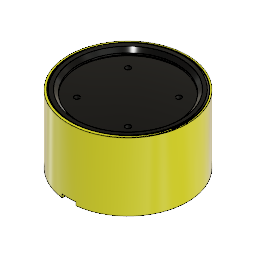
Rotating ROV thruster base v10 (Autodesk Fusion 360 archive; units mm, degrees)
design "Rotating ROV thruster base" references "Servo sg90"
Autodesk Fusion 360 part; units mm, degrees
note: some values were not read from the file. Set by a fixed rule: which face or edge a step refers to.
sketch "Sketch1" plane through (0, 0, 0) normal (0, 0, 1) x (1, 0, 0)
  line L0 (-15, 15) -> (15, 15) construction
  line L1 (15, 15) -> (15, -15) construction
  line L2 (15, -15) -> (-15, -15) construction
  line L3 (-15, -15) -> (-15, 15) construction
  line L4 (-15, 15) -> (15, -15) construction
  line L5 (15, 15) -> (-15, -15) construction
  circle A0 centre (15, 15) radius 1.5
  circle A1 centre (-15, 15) radius 1.5
  circle A2 centre (-15, -15) radius 1.5
  circle A3 centre (15, -15) radius 1.5
  line L6 (-20, 20) -> (20, 20)
  line L7 (20, 20) -> (20, -20)
  line L8 (20, -20) -> (-20, -20)
  line L9 (-20, -20) -> (-20, 20)
  line L10 (-20, 20) -> (20, -20) construction
  line L11 (20, 20) -> (-20, -20) construction
  circle A4 centre (-15, 15) radius 3
  circle A5 centre (15, 15) radius 3
  circle A6 centre (-15, -15) radius 3
  circle A7 centre (15, -15) radius 3
  circle A8 centre (0, 0) radius 35
  dimension "d1" = 30
  dimension "d2" = 30
  dimension "d3" = 3
  dimension "d4" = 3
  dimension "d5" = 3
  dimension "d6" = 3
  dimension "d7" = 40
  dimension "d8" = 40
  dimension "d11" = 6
  dimension "d12" = 6
  dimension "d13" = 6
  dimension "d14" = 6
  constraint perpendicular L0 L1
  constraint parallel L0 L2
  constraint parallel L1 L3
  constraint horizontal L0
  constraint coincident L4 A8.centre
  constraint coincident L5 A8.centre
  constraint coincident A8.centre origin
  constraint coincident L0.end L1.start
  constraint coincident L0.start L3.end
  constraint coincident L2.end L3.start
  constraint coincident L1.end L2.start
  constraint perpendicular L6 L7
  constraint parallel L6 L8
  constraint parallel L7 L9
  constraint horizontal L6
  constraint coincident L10 A8.centre
  constraint coincident L11 A8.centre
  constraint concentric A1 A4
  constraint concentric A0 A5
  constraint concentric A2 A6
  constraint concentric A3 A7
  measures "d1" distance of L0.end L1.end
  measures "d2" distance of L1.end L2.end
  measures "d3" diameter of A0
  measures "d4" diameter of A1
  measures "d5" diameter of A2
  measures "d6" diameter of A3
  measures "d7" distance of L7.end L8.end
  measures "d8" distance of L6.end L7.end
  measures "d11" diameter of A4
  measures "d12" diameter of A5
  measures "d13" diameter of A6
  measures "d14" diameter of A7
extrude "Extrude3" add sketch "Sketch1" along normal blind 16 contours L6 L7 L8 L9 makes body 1
extrude "Extrude4" add sketch "Sketch1" along normal blind 2 contours A4 | A5 | A6 | A7 bodies 1
sketch "Sketch2" plane through (0, 0, 16) normal (0, 0, 1) x (-1, 0, 0)
  circle A0 centre (15, 15) radius 3
  circle A1 centre (-15, -15) radius 3
  circle A2 centre (-15, 15) radius 3
  circle A3 centre (15, -15) radius 3
  line L0 (20, 20) -> (-20, 20)
  line L1 (-20, 20) -> (-20, -20)
  line L2 (-20, -20) -> (20, -20)
  line L3 (20, -20) -> (20, 20)
  line L4 (6.225, 16.425) -> (-6.225, 16.425)
  line L5 (-6.225, 16.425) -> (-6.225, -6.425)
  line L6 (-6.225, -6.425) -> (6.225, -6.425)
  line L7 (6.225, -6.425) -> (6.225, 16.425)
  circle A4 centre (0, -8.925) radius 1.5
  line L8 (-20, 0) -> (-2.5, 0)
  line L9 (-6.225, 5) -> (6.225, 5) construction
  circle A5 centre (0, 18.925) radius 1.5
  dimension "d21" = 12.45
  dimension "d22" = 22.85
  dimension "d25" = 3
  constraint perpendicular L4 L5
  constraint parallel L4 L6
  constraint parallel L5 L7
  constraint horizontal L4
  constraint midpoint L5 L9.start
  constraint midpoint L7 L9.end
  constraint symmetric A4 L9 A5
  measures "d21" distance of L5.end L6.end
  measures "d22" distance of L4.end L5.end
  measures "d25" diameter of A4
extrude "Extrude5" cut sketch "Sketch2" against normal up to surface (16 mm away) contours L4 L5 L6 L7 bodies 1
sketch "Sketch3" plane through (0, 20, 0) normal (0, 1, 0) x (-1, 0, 0)
  line L0 (-20, 0) -> (20, 0)
  line L1 (20, 0) -> (20, 16)
  line L2 (20, 16) -> (-20, 16)
  line L3 (-20, 16) -> (-20, 0)
  line L4 (-4, 2) -> (4, 2)
  line L5 (4, 2) -> (4, -2)
  line L6 (4, -2) -> (-4, -2)
  line L7 (-4, -2) -> (-4, 2)
  line L8 (-4, 2) -> (4, -2) construction
  line L9 (4, 2) -> (-4, -2) construction
  constraint perpendicular L4 L5
  constraint parallel L4 L6
  constraint parallel L5 L7
  constraint horizontal L4
  constraint coincident L8 origin
  constraint coincident L9 origin
extrude "Extrude7" cut sketch "Sketch2" against normal blind 10 contours L0 A5 | L0 A5 | A4 bodies 1
extrude "Extrude8" add sketch "Sketch1" along normal blind 16 contours A8 bodies 1
extrude "Extrude6" cut sketch "Sketch3" along normal blind 30 and the other way blind 65 contours L0 L4 L5 L7 bodies 1
sketch "Sketch4" plane through (0, 0, 16) normal (0, 0, 1) x (-1, 0, 0)
  circle A0 centre (0, 0) radius 35
  circle A1 centre (0, -8.925) radius 1.5
  line L0 (6.225, -6.425) -> (-6.225, -6.425)
  line L1 (-6.225, -6.425) -> (-6.225, 16.425)
  line L2 (-6.225, 16.425) -> (6.225, 16.425)
  line L3 (6.225, 16.425) -> (6.225, -6.425)
  circle A2 centre (15, 15) radius 3
  circle A3 centre (-15, 15) radius 3
  circle A4 centre (-15, -15) radius 3
  circle A5 centre (15, -15) radius 3
  circle A6 centre (0, 0) radius 33
  arc A7 (-1.0461, 20) -> (1.0461, 20) centre (0, 18.925) ccw
  line L4 (-1.0461, 20) -> (1.0461, 20)
  dimension "d34" = -2
extrude "Extrude9" add sketch "Sketch4" along normal blind 20 contours A0 bodies 1
sketch "Sketch6" plane through (0, 0, 16) normal (0, 0, 1) x (-1, 0, 0)
  circle A0 centre (0, 0) radius 33
  circle A1 centre (0, -8.925) radius 1.5
  line L0 (6.225, -6.425) -> (-6.225, -6.425)
  line L1 (-6.225, -6.425) -> (-6.225, 16.425)
  line L2 (-6.225, 16.425) -> (6.225, 16.425)
  line L3 (6.225, 16.425) -> (6.225, -6.425)
  circle A2 centre (15, 15) radius 3
  circle A3 centre (-15, 15) radius 3
  circle A4 centre (-15, -15) radius 3
  circle A5 centre (15, -15) radius 3
  line L4 (6.225, -11.775) -> (-6.225, -11.775)
  line L5 (-6.225, -11.775) -> (-6.225, 20.475)
  line L6 (-6.225, 20.475) -> (6.225, 20.475)
  line L7 (6.225, 20.475) -> (6.225, -11.775)
  arc A6 (-1.0461, 20) -> (1.0461, 20) centre (0, 18.925) ccw
  line L8 (-1.0461, 20) -> (1.0461, 20)
  point P0 (6.225, -11.775)
  point P1 (-6.225, 20.475)
  constraint horizontal L4
  constraint vertical L5
  constraint horizontal L6
  constraint vertical L7
  constraint coincident P1 L5.end
  constraint coincident P0 L4.start
extrude "Extrude11" add sketch "Sketch6" along normal blind 11 contours A0 bodies 1
sketch "Sketch8" plane through (0, 0, 27) normal (0, 0, 1) x (-1, 0, 0)
  circle A0 centre (15, -15) radius 3
  circle A1 centre (-15, 15) radius 3
  circle A2 centre (-15, -15) radius 3
  line L0 (-6.225, 20.475) -> (6.225, 20.475)
  line L1 (6.225, 20.475) -> (6.225, -11.775)
  line L2 (6.225, -11.775) -> (-6.225, -11.775)
  line L3 (-6.225, -11.775) -> (-6.225, 20.475)
  circle A3 centre (15, 15) radius 3
  circle A4 centre (0, 0) radius 33
  circle A5 centre (0, 0) radius 30
  line L4 (13.2679, -12) -> (11.5359, -15)
  line L5 (11.5359, -15) -> (13.2679, -18)
  line L6 (13.2679, -18) -> (16.7321, -18)
  line L7 (16.7321, -18) -> (18.4641, -15)
  line L8 (18.4641, -15) -> (16.7321, -12)
  line L9 (16.7321, -12) -> (13.2679, -12)
  line L10 (-16.7321, -12) -> (-18.4641, -15)
  line L11 (-18.4641, -15) -> (-16.7321, -18)
  line L12 (-16.7321, -18) -> (-13.2679, -18)
  line L13 (-13.2679, -18) -> (-11.5359, -15)
  line L14 (-11.5359, -15) -> (-13.2679, -12)
  line L15 (-13.2679, -12) -> (-16.7321, -12)
  line L16 (-16.7321, 18) -> (-18.4641, 15)
  line L17 (-18.4641, 15) -> (-16.7321, 12)
  line L18 (-16.7321, 12) -> (-13.2679, 12)
  line L19 (-13.2679, 12) -> (-11.5359, 15)
  line L20 (-11.5359, 15) -> (-13.2679, 18)
  line L21 (-13.2679, 18) -> (-16.7321, 18)
  line L22 (13.2679, 18) -> (11.5359, 15)
  line L23 (11.5359, 15) -> (13.2679, 12)
  line L24 (13.2679, 12) -> (16.7321, 12)
  line L25 (16.7321, 12) -> (18.4641, 15)
  line L26 (18.4641, 15) -> (16.7321, 18)
  line L27 (16.7321, 18) -> (13.2679, 18)
  point P0 (15, -15)
  point P1 (-15, -15)
  point P2 (-15, 15)
  point P3 (15, 15)
  dimension "d44" = -3
  constraint coincident P0 A0.centre
  constraint coincident P1 A2.centre
  constraint coincident A1.centre P2
  constraint coincident P3 A3.centre
extrude "Extrude12" add sketch "Sketch8" along normal blind 5 separate body contours A5 makes body 2
sketch "Sketch9" plane through (0, 0, 32) normal (0, 0, 1) x (-1, 0, 0)
  line L0 (6.225, -11.775) -> (-6.225, -11.775)
  line L1 (-6.225, -11.775) -> (-6.225, 20.475)
  line L2 (-6.225, 20.475) -> (6.225, 20.475)
  line L3 (6.225, 20.475) -> (6.225, -11.775)
  circle A0 centre (0, 0) radius 30
  circle A1 centre (-15, -15) radius 1.5
  circle A2 centre (15, -15) radius 1.5
  circle A3 centre (15, 15) radius 1.5
  circle A4 centre (-15, 15) radius 1.5
  line L4 (13.2679, 18) -> (16.7321, 18)
  line L5 (16.7321, 18) -> (18.4641, 15)
  line L6 (18.4641, 15) -> (16.7321, 12)
  line L7 (16.7321, 12) -> (13.2679, 12)
  line L8 (13.2679, 12) -> (11.5359, 15)
  line L9 (11.5359, 15) -> (13.2679, 18)
  line L10 (-16.7321, -12) -> (-13.2679, -12)
  line L11 (-13.2679, -12) -> (-11.5359, -15)
  line L12 (-11.5359, -15) -> (-13.2679, -18)
  line L13 (-13.2679, -18) -> (-16.7321, -18)
  line L14 (-16.7321, -18) -> (-18.4641, -15)
  line L15 (-18.4641, -15) -> (-16.7321, -12)
  line L16 (-16.7321, 18) -> (-13.2679, 18)
  line L17 (-13.2679, 18) -> (-11.5359, 15)
  line L18 (-11.5359, 15) -> (-13.2679, 12)
  line L19 (-13.2679, 12) -> (-16.7321, 12)
  line L20 (-16.7321, 12) -> (-18.4641, 15)
  line L21 (-18.4641, 15) -> (-16.7321, 18)
  line L22 (13.2679, -12) -> (16.7321, -12)
  line L23 (16.7321, -12) -> (18.4641, -15)
  line L24 (18.4641, -15) -> (16.7321, -18)
  line L25 (16.7321, -18) -> (13.2679, -18)
  line L26 (13.2679, -18) -> (11.5359, -15)
  line L27 (11.5359, -15) -> (13.2679, -12)
extrude "Extrude13" add sketch "Sketch9" along normal blind 4 contours A0 | L4 L5 L6 L7 L8 L9 | L10 L11 L12 L13 L14 L15 | L16 L17 L18 L19 L20 L21 | L22 L23 L24 L25 L26 L27 bodies 2
sketch "Sketch10" plane through (0, 0, 31) normal (0, 0, 1) x (-1, 0, 0)
  arc A0 (-0.3428, -2.4361) -> (-0.3241, -2.4389) centre (0, -0.225) ccw
  arc A1 (-0.3241, -2.4389) -> (0.3241, -2.4389) centre (0, -2.4625) ccw
  arc A2 (0.3241, -2.4389) -> (0.3428, -2.4361) centre (0, -0.225) ccw
  arc A3 (0.3428, -2.4361) -> (0.9623, -2.245) centre (0.6595, -2.3631) ccw
  arc A4 (0.9623, -2.245) -> (0.9793, -2.2368) centre (0, -0.225) ccw
  arc A5 (0.9793, -2.2368) -> (1.515, -1.8716) centre (1.2604, -2.0737) ccw
  arc A6 (1.515, -1.8716) -> (1.5288, -1.8588) centre (0, -0.225) ccw
  arc A7 (1.5288, -1.8588) -> (1.933, -1.3519) centre (1.7493, -1.6201) ccw
  arc A8 (1.933, -1.3519) -> (1.9424, -1.3356) centre (0, -0.225) ccw
  arc A9 (1.9424, -1.3356) -> (2.1793, -0.7321) centre (2.0828, -1.0425) ccw
  arc A10 (2.1793, -0.7321) -> (2.1835, -0.7137) centre (0, -0.225) ccw
  arc A11 (2.1835, -0.7137) -> (2.2319, -0.0672) centre (2.2312, -0.3922) ccw
  arc A12 (2.2319, -0.0672) -> (2.2305, -0.0484) centre (0, -0.225) ccw
  arc A13 (2.2305, -0.0484) -> (2.0863, 0.5837) centre (2.1814, 0.2729) ccw
  arc A14 (2.0863, 0.5837) -> (2.0794, 0.6012) centre (0, -0.225) ccw
  arc A15 (2.0794, 0.6012) -> (1.7552, 1.1627) centre (1.9377, 0.8938) ccw
  arc A16 (1.7552, 1.1627) -> (1.7434, 1.1774) centre (0, -0.225) ccw
  arc A17 (1.7434, 1.1774) -> (1.2682, 1.6184) centre (1.5219, 1.4152) ccw
  arc A18 (1.2682, 1.6184) -> (1.2526, 1.629) centre (0, -0.225) ccw
  arc A19 (1.2526, 1.629) -> (0.6685, 1.9103) centre (0.9708, 1.7909) ccw
  arc A20 (0.6685, 1.9103) -> (0.6505, 1.9159) centre (0, -0.225) ccw
  arc A21 (0.6505, 1.9159) -> (0.0094, 2.0125) centre (0.3335, 1.9875) ccw
  arc A22 (0.0094, 2.0125) -> (-0.0094, 2.0125) centre (0, -0.225) ccw
  arc A23 (-0.0094, 2.0125) -> (-0.6505, 1.9159) centre (-0.3335, 1.9875) ccw
  arc A24 (-0.6505, 1.9159) -> (-0.6685, 1.9103) centre (0, -0.225) ccw
  arc A25 (-0.6685, 1.9103) -> (-1.2526, 1.629) centre (-0.9708, 1.7909) ccw
  arc A26 (-1.2526, 1.629) -> (-1.2682, 1.6184) centre (0, -0.225) ccw
  arc A27 (-1.2682, 1.6184) -> (-1.7434, 1.1774) centre (-1.5219, 1.4152) ccw
  arc A28 (-1.7434, 1.1774) -> (-1.7552, 1.1627) centre (0, -0.225) ccw
  arc A29 (-1.7552, 1.1627) -> (-2.0794, 0.6012) centre (-1.9377, 0.8938) ccw
  arc A30 (-2.0794, 0.6012) -> (-2.0863, 0.5837) centre (0, -0.225) ccw
  arc A31 (-2.0863, 0.5837) -> (-2.2305, -0.0484) centre (-2.1814, 0.2729) ccw
  arc A32 (-2.2305, -0.0484) -> (-2.2319, -0.0672) centre (0, -0.225) ccw
  arc A33 (-2.2319, -0.0672) -> (-2.1835, -0.7137) centre (-2.2312, -0.3922) ccw
  arc A34 (-2.1835, -0.7137) -> (-2.1793, -0.7321) centre (0, -0.225) ccw
  arc A35 (-2.1793, -0.7321) -> (-1.9424, -1.3356) centre (-2.0828, -1.0425) ccw
  arc A36 (-1.9424, -1.3356) -> (-1.933, -1.3519) centre (0, -0.225) ccw
  arc A37 (-1.933, -1.3519) -> (-1.5288, -1.8588) centre (-1.7493, -1.6201) ccw
  arc A38 (-1.5288, -1.8588) -> (-1.515, -1.8716) centre (0, -0.225) ccw
  arc A39 (-1.515, -1.8716) -> (-0.9793, -2.2368) centre (-1.2604, -2.0737) ccw
  arc A40 (-0.9793, -2.2368) -> (-0.9623, -2.245) centre (0, -0.225) ccw
  arc A41 (-0.9623, -2.245) -> (-0.3428, -2.4361) centre (-0.6595, -2.3631) ccw
  line L0 (-6.225, -11.775) -> (6.225, -11.775)
  line L1 (6.225, -11.775) -> (6.225, 20.475)
  line L2 (6.225, 20.475) -> (-6.225, 20.475)
  line L3 (-6.225, 20.475) -> (-6.225, -11.775)
  arc A42 (-0.7462, 1.778) -> (-1.1008, 1.6073) centre (-0.9708, 1.7909) ccw
  arc A43 (-1.1008, 1.6073) -> (-1.3034, 1.4691) centre (0, -0.225) ccw
  arc A44 (-1.3034, 1.4691) -> (-1.592, 1.2014) centre (-1.5219, 1.4152) ccw
  arc A45 (-1.592, 1.2014) -> (-1.7449, 1.0096) centre (0, -0.225) ccw
  arc A46 (-1.7449, 1.0096) -> (-1.9417, 0.6688) centre (-1.9377, 0.8938) ccw
  arc A47 (-1.9417, 0.6688) -> (-2.0313, 0.4405) centre (0, -0.225) ccw
  arc A48 (-2.0313, 0.4405) -> (-2.1188, 0.0568) centre (-2.1814, 0.2729) ccw
  arc A49 (-2.1188, 0.0568) -> (-2.1372, -0.1878) centre (0, -0.225) ccw
  arc A50 (-2.1372, -0.1878) -> (-2.1078, -0.5803) centre (-2.2312, -0.3922) ccw
  arc A51 (-2.1078, -0.5803) -> (-2.0532, -0.8194) centre (0, -0.225) ccw
  arc A52 (-2.0532, -0.8194) -> (-1.9094, -1.1858) centre (-2.0828, -1.0425) ccw
  arc A53 (-1.9094, -1.1858) -> (-1.7868, -1.3982) centre (0, -0.225) ccw
  arc A54 (-1.7868, -1.3982) -> (-1.5414, -1.7059) centre (-1.7493, -1.6201) ccw
  arc A55 (-1.5414, -1.7059) -> (-1.3616, -1.8727) centre (0, -0.225) ccw
  arc A56 (-1.3616, -1.8727) -> (-1.0364, -2.0944) centre (-1.2604, -2.0737) ccw
  arc A57 (-1.0364, -2.0944) -> (-0.8154, -2.2009) centre (0, -0.225) ccw
  arc A58 (-0.8154, -2.2009) -> (-0.4393, -2.3169) centre (-0.6595, -2.3631) ccw
  arc A59 (-0.4393, -2.3169) -> (-0.1968, -2.3534) centre (0, -0.225) ccw
  arc A60 (-0.1968, -2.3534) -> (0.1968, -2.3534) centre (0, -2.4625) ccw
  arc A61 (0.1968, -2.3534) -> (0.4393, -2.3169) centre (0, -0.225) ccw
  arc A62 (0.4393, -2.3169) -> (0.8154, -2.2009) centre (0.6595, -2.3631) ccw
  arc A63 (0.8154, -2.2009) -> (1.0364, -2.0944) centre (0, -0.225) ccw
  arc A64 (1.0364, -2.0944) -> (1.3616, -1.8727) centre (1.2604, -2.0737) ccw
  arc A65 (1.3616, -1.8727) -> (1.5414, -1.7059) centre (0, -0.225) ccw
  arc A66 (1.5414, -1.7059) -> (1.7868, -1.3982) centre (1.7493, -1.6201) ccw
  arc A67 (1.7868, -1.3982) -> (1.9094, -1.1858) centre (0, -0.225) ccw
  arc A68 (1.9094, -1.1858) -> (2.0532, -0.8194) centre (2.0828, -1.0425) ccw
  arc A69 (2.0532, -0.8194) -> (2.1078, -0.5803) centre (0, -0.225) ccw
  arc A70 (2.1078, -0.5803) -> (2.1372, -0.1878) centre (2.2312, -0.3922) ccw
  arc A71 (2.1372, -0.1878) -> (2.1188, 0.0568) centre (0, -0.225) ccw
  arc A72 (2.1188, 0.0568) -> (2.0313, 0.4405) centre (2.1814, 0.2729) ccw
  arc A73 (2.0313, 0.4405) -> (1.9417, 0.6688) centre (0, -0.225) ccw
  arc A74 (1.9417, 0.6688) -> (1.7449, 1.0096) centre (1.9377, 0.8938) ccw
  arc A75 (1.7449, 1.0096) -> (1.592, 1.2014) centre (0, -0.225) ccw
  arc A76 (1.592, 1.2014) -> (1.3034, 1.4691) centre (1.5219, 1.4152) ccw
  arc A77 (1.3034, 1.4691) -> (1.1008, 1.6073) centre (0, -0.225) ccw
  arc A78 (1.1008, 1.6073) -> (0.7462, 1.778) centre (0.9708, 1.7909) ccw
  arc A79 (0.7462, 1.778) -> (0.5118, 1.8503) centre (0, -0.225) ccw
  arc A80 (0.5118, 1.8503) -> (0.1226, 1.909) centre (0.3335, 1.9875) ccw
  arc A81 (0.1226, 1.909) -> (-0.1226, 1.909) centre (0, -0.225) ccw
  arc A82 (-0.1226, 1.909) -> (-0.5118, 1.8503) centre (-0.3335, 1.9875) ccw
  arc A83 (-0.5118, 1.8503) -> (-0.7462, 1.778) centre (0, -0.225) ccw
  point P0 (-6.225, -11.775)
  point P1 (6.225, 20.475)
  dimension "d49" = -0.1
  constraint horizontal L0
  constraint vertical L1
  constraint horizontal L2
  constraint vertical L3
  constraint coincident P1 L1.end
  constraint coincident P0 L0.start
extrude "Extrude14" add sketch "Sketch10" against normal blind 4 contours A0 A1 A2 A3 A4 A5 A6 A7 A8 A9 A10 A11 A12 A13 A14 A15 A16 A17 A18 A19 A20 A21 A22 A23 A24 A25 A26 A27 A28 A29 A30 A31 A32 A33 A34 A35 A36 A37 A38 A39 A40 A41 | L0 L1 L2 L3 bodies 2
sketch "Sketch11" plane through (0, 0, 31) normal (0, 0, 1) x (-1, 0, 0)
  arc A0 (-0.1226, 1.909) -> (-0.5118, 1.8503) centre (-0.3335, 1.9875) ccw
  arc A1 (0.5118, 1.8503) -> (0.1226, 1.909) centre (0.3335, 1.9875) ccw
  arc A2 (1.1008, 1.6073) -> (0.7462, 1.778) centre (0.9708, 1.7909) ccw
  arc A3 (1.592, 1.2014) -> (1.3034, 1.4691) centre (1.5219, 1.4152) ccw
  arc A4 (1.9417, 0.6688) -> (1.7449, 1.0096) centre (1.9377, 0.8937) ccw
  arc A5 (2.1188, 0.0568) -> (2.0313, 0.4405) centre (2.1814, 0.2729) ccw
  arc A6 (2.1078, -0.5803) -> (2.1372, -0.1878) centre (2.2312, -0.3922) ccw
  arc A7 (1.9094, -1.1858) -> (2.0532, -0.8194) centre (2.0828, -1.0425) ccw
  arc A8 (1.5414, -1.7059) -> (1.7868, -1.3982) centre (1.7493, -1.6201) ccw
  arc A9 (1.0364, -2.0944) -> (1.3616, -1.8727) centre (1.2604, -2.0737) ccw
  arc A10 (0.4393, -2.3169) -> (0.8154, -2.2009) centre (0.6595, -2.3631) ccw
  arc A11 (-0.1968, -2.3534) -> (0.1968, -2.3534) centre (0, -2.4625) ccw
  arc A12 (-0.8154, -2.2009) -> (-0.4393, -2.3169) centre (-0.6595, -2.3631) ccw
  arc A13 (-1.3616, -1.8727) -> (-1.0364, -2.0944) centre (-1.2604, -2.0737) ccw
  arc A14 (-1.7868, -1.3982) -> (-1.5414, -1.7059) centre (-1.7493, -1.6201) ccw
  arc A15 (-2.0532, -0.8194) -> (-1.9094, -1.1858) centre (-2.0828, -1.0425) ccw
  arc A16 (-2.1372, -0.1878) -> (-2.1078, -0.5803) centre (-2.2312, -0.3922) ccw
  arc A17 (-2.0313, 0.4405) -> (-2.1188, 0.0568) centre (-2.1814, 0.2729) ccw
  arc A18 (-1.7449, 1.0096) -> (-1.9417, 0.6688) centre (-1.9377, 0.8937) ccw
  arc A19 (-1.3034, 1.4691) -> (-1.592, 1.2014) centre (-1.5219, 1.4152) ccw
  arc A20 (-0.7462, 1.778) -> (-1.1008, 1.6073) centre (-0.9708, 1.7909) ccw
  line L0 (-6.225, 20.475) -> (-6.225, -11.775)
  line L1 (-6.225, -11.775) -> (6.225, -11.775)
  line L2 (6.225, -11.775) -> (6.225, 20.475)
  line L3 (6.225, 20.475) -> (-6.225, 20.475)
  line L4 (8, -13) -> (-7, -13)
  line L5 (-7, -13) -> (-7, 21)
  line L6 (-7, 21) -> (8, 21)
  line L7 (8, 21) -> (8, -13)
  arc A21 (-0.5118, 1.8503) -> (-0.7462, 1.778) centre (0, -0.225) ccw
  arc A22 (0.1226, 1.909) -> (-0.1226, 1.909) centre (0, -0.225) ccw
  arc A23 (0.7462, 1.778) -> (0.5118, 1.8503) centre (0, -0.225) ccw
  arc A24 (1.3034, 1.4691) -> (1.1008, 1.6073) centre (0, -0.225) ccw
  arc A25 (1.7449, 1.0096) -> (1.592, 1.2014) centre (0, -0.225) ccw
  arc A26 (2.0313, 0.4405) -> (1.9417, 0.6688) centre (0, -0.225) ccw
  arc A27 (2.1372, -0.1878) -> (2.1188, 0.0568) centre (0, -0.225) ccw
  arc A28 (2.0532, -0.8194) -> (2.1078, -0.5803) centre (0, -0.225) ccw
  arc A29 (1.7868, -1.3982) -> (1.9094, -1.1858) centre (0, -0.225) ccw
  arc A30 (1.3616, -1.8727) -> (1.5414, -1.7059) centre (0, -0.225) ccw
  arc A31 (0.8154, -2.2009) -> (1.0364, -2.0944) centre (0, -0.225) ccw
  arc A32 (0.1968, -2.3534) -> (0.4393, -2.3169) centre (0, -0.225) ccw
  arc A33 (-0.4393, -2.3169) -> (-0.1968, -2.3534) centre (0, -0.225) ccw
  arc A34 (-1.0364, -2.0944) -> (-0.8154, -2.2009) centre (0, -0.225) ccw
  arc A35 (-1.5414, -1.7059) -> (-1.3616, -1.8727) centre (0, -0.225) ccw
  arc A36 (-1.9094, -1.1858) -> (-1.7868, -1.3982) centre (0, -0.225) ccw
  arc A37 (-2.1078, -0.5803) -> (-2.0532, -0.8194) centre (0, -0.225) ccw
  arc A38 (-2.1188, 0.0568) -> (-2.1372, -0.1878) centre (0, -0.225) ccw
  arc A39 (-1.9417, 0.6688) -> (-2.0313, 0.4405) centre (0, -0.225) ccw
  arc A40 (-1.592, 1.2014) -> (-1.7449, 1.0096) centre (0, -0.225) ccw
  arc A41 (-1.1008, 1.6073) -> (-1.3034, 1.4691) centre (0, -0.225) ccw
  constraint horizontal L4
  constraint vertical L5
  constraint horizontal L6
  constraint vertical L7
extrude "Extrude15" add sketch "Sketch11" along normal blind 5 contours A0 A1 A2 A3 A4 A5 A6 A7 A8 A9 A10 A11 A12 A13 A14 A15 A16 A17 A18 A19 A20 A21 A22 A23 A24 A25 A26 A27 A28 A29 A30 A31 A32 A33 A34 A35 A36 A37 A38 A39 A40 A41 | L0 L1 L2 L3 bodies 2
sketch "Sketch12" plane through (0, 0, 36) normal (0, 0, 1) x (-1, 0, 0)
  circle A0 centre (0, 0) radius 33
  circle A1 centre (0, 0) radius 35
  circle A2 centre (0, 0) radius 34.2
  dimension "d54" = -0.8
extrude "Extrude16" add sketch "Sketch12" along normal blind 4 contours A1 bodies 1
extrude "Extrude18" cut 1 faces at (-33.5498, 3.3385, 36) along direction (0, 0, -1) blind 9 on bodies 1 bodies 1
thread "Thread1" "ISO Metric profile 68.0 M68x1.5 6H" major diameter 68.2143 minor diameter 66.5262 pitch 1.5 angle 60 modelled right hand crest width 0.1875 on face at (-34.0301, 3.4052, 37.3333) from (0, 0, 36) to (0, 0, 40) crest through (-33.2631, 0, 26.1562) on bodies 1
sketch "Sketch13" plane through (0, 0, 36) normal (0, 0, 1) x (-1, 0, 0)
  circle A0 centre (15, 15) radius 1.5
  circle A1 centre (15, -15) radius 1.5
  circle A2 centre (-15, 15) radius 1.5
  circle A3 centre (-15, -15) radius 1.5
  circle A4 centre (0, 0) radius 30
  circle A5 centre (0, 0) radius 29
  circle A6 centre (0, 0) radius 30
  dimension "d57" = 58
  dimension "d58" = 1
  constraint coincident A4.centre A5.centre
  measures "d57" diameter of A5
extrude "Extrude17" add sketch "Sketch13" along normal blind 4 and the other way blind -1 separate body contours A4 A6 makes body 3
thread "Thread2" "ISO Metric profile 68.0 M68x1.5 6g" major diameter 67.85 minor diameter 66.1269 pitch 1.5 angle 60 modelled right hand crest width 0.1875 on face at (-29.8509, 2.987, 38) crest through (-33.925, 0, 36.9062) on bodies 3
chamfer "Chamfer1" distance 2 angle 45 1 edges at (27.0375, -10.4868, 40) on bodies 3
chamfer "Chamfer2" distance 3 angle 45 4 edges at (0, 11.775, 27) (-6.225, -4.35, 27) (6.225, -4.35, 27) (0, -20.475, 27) on bodies 1
chamfer "Chamfer3" distance 2 angle 45 4 edges at (6.225, -4.35, 24) (0, -20.475, 24) (-6.225, -4.35, 24) (0, 11.775, 24) on bodies 1
move_body "Move1" bodies 3 to x (1, 0, 0) y (0, 1, 0) z (0, 0, 1) at (0, 0, 0.1)

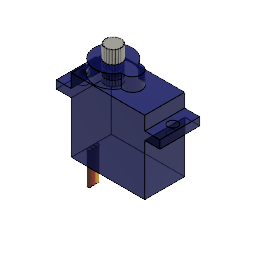
design "Servo sg90"
Autodesk Fusion 360 part; units mm, degrees
sketch "Sketch1" plane through (0, 0, 0) normal (0, 0, 1) x (1, 0, 0)
  line L0 (-11.425, 6.225) -> (11.425, 6.225)
  line L1 (11.425, 6.225) -> (11.425, -6.225)
  line L2 (11.425, -6.225) -> (-11.425, -6.225)
  line L3 (-11.425, -6.225) -> (-11.425, 6.225)
  line L4 (-11.425, 6.225) -> (11.425, -6.225) construction
  line L5 (11.425, 6.225) -> (-11.425, -6.225) construction
  line L6 (-16.125, 6.225) -> (16.125, 6.225)
  line L7 (16.125, 6.225) -> (16.125, -6.225)
  line L8 (16.125, -6.225) -> (-16.125, -6.225)
  line L9 (-16.125, -6.225) -> (-16.125, 6.225)
  line L10 (-16.125, 6.225) -> (16.125, -6.225) construction
  line L11 (16.125, 6.225) -> (-16.125, -6.225) construction
  circle A0 centre (-10.85, 0) radius 0.575
  line L12 (-10.85, 0) -> (-10.85, -1.15) construction
  line L13 (-10.85, 0) -> (-10.85, 1.15) construction
  circle A1 centre (-10.85, -1.15) radius 0.575
  circle A2 centre (-10.85, 1.15) radius 0.575
  dimension "d1" = 22.85
  dimension "d2" = 12.45
  dimension "d5" = 32.25
  dimension "d6" = 12.45
  dimension "d31" = 1.15
  dimension "d32" = 1.15
  dimension "d33" = 1.15
  dimension "d34" = 1.15
  dimension "d35" = 1.15
  constraint perpendicular L0 L1
  constraint parallel L0 L2
  constraint parallel L1 L3
  constraint horizontal L0
  constraint coincident L4 origin
  constraint coincident L5 origin
  constraint perpendicular L6 L7
  constraint parallel L6 L8
  constraint parallel L7 L9
  constraint horizontal L6
  constraint coincident L10 origin
  constraint coincident L11 origin
  constraint coincident A0.centre L12.start
  constraint vertical L12
  constraint parallel L12 L13
  constraint coincident L12.end A1.centre
  constraint coincident L13.end A2.centre
  measures "d1" distance of L1.end L2.end
  measures "d2" distance of L0.end L1.end
  measures "d5" distance of L7.end L8.end
  measures "d6" distance of L6.end L7.end
  measures "d31" diameter of A0
  measures "d32" distance of A0.centre L12.end
  measures "d33" distance of A0.centre L13.end
  measures "d34" diameter of A1
  measures "d35" diameter of A2
extrude "Extrude7" add sketch "Sketch1" against normal blind 10 contours A2 | A0 | A1 makes body 1
extrude "Extrude1" add sketch "Sketch1" along normal blind 22.75 separate body contours L0 L1 L2 L3 L6 L8 A0 A1 A2 | L3 A0 A2 | A2 | L3 A0 A1 | A0 | A1 makes body 2
extrude "Extrude2" add sketch "Sketch1" along normal blind 16 and the other way blind -18.5 contours L3 L6 L8 L9 | L1 L6 L7 L8 bodies 2
sketch "Sketch2" plane through (0, 0, 18.5) normal (0, 0, 1) x (-1, 0, 0)
  line L0 (11.425, 6.225) -> (11.425, -6.225)
  line L1 (11.425, -6.225) -> (16.125, -6.225)
  line L2 (16.125, -6.225) -> (16.125, 6.225)
  line L3 (16.125, 6.225) -> (11.425, 6.225)
  line L4 (11.425, 0) -> (12.425, 0) construction
  circle A0 centre (13.925, 0) radius 1.5
  line L5 (0, 0) -> (0, -3)
  circle A1 centre (-13.925, 0) radius 1.5
  dimension "d11" = 1
  dimension "d12" = 3
  constraint midpoint L0 L4.start
  constraint perpendicular L0 L4
  constraint coincident L4.end A0
  constraint coincident L5.start origin
  constraint vertical L5
  constraint symmetric A0 L5 A1
  measures "d11" distance of L4.start L4.end
  measures "d12" diameter of A0
extrude "Extrude3" cut sketch "Sketch2" against normal blind 6 contours A0 | A1 bodies 2
sketch "Sketch3" plane through (0, 0, 22.75) normal (0, 0, 1) x (-1, 0, 0)
  line L0 (11.425, 6.225) -> (-11.425, 6.225)
  line L1 (-11.425, 6.225) -> (-11.425, -6.225)
  line L2 (-11.425, -6.225) -> (11.425, -6.225)
  line L3 (11.425, -6.225) -> (11.425, 6.225)
  line L4 (-11.425, 0) -> (4.575, 0) construction
  circle A0 centre (4.575, 0) radius 5.875
  circle A1 centre (4.575, 0) radius 2.2375
  circle A2 centre (6.8125, 0) radius 0.325
  circle A3 centre (6.7131, 0.6595) radius 0.325
  circle A4 centre (6.4237, 1.2604) radius 0.325
  circle A5 centre (5.9701, 1.7493) radius 0.325
  circle A6 centre (5.3925, 2.0828) radius 0.325
  circle A7 centre (4.7422, 2.2312) radius 0.325
  circle A8 centre (4.0771, 2.1814) radius 0.325
  circle A9 centre (3.4562, 1.9377) radius 0.325
  circle A10 centre (2.9348, 1.5219) radius 0.325
  circle A11 centre (2.5591, 0.9708) radius 0.325
  circle A12 centre (2.3625, 0.3335) radius 0.325
  circle A13 centre (2.3625, -0.3335) radius 0.325
  circle A14 centre (2.5591, -0.9708) radius 0.325
  circle A15 centre (2.9348, -1.5219) radius 0.325
  circle A16 centre (3.4563, -1.9377) radius 0.325
  circle A17 centre (4.0771, -2.1814) radius 0.325
  circle A18 centre (4.7422, -2.2312) radius 0.325
  circle A19 centre (5.3925, -2.0828) radius 0.325
  circle A20 centre (5.9701, -1.7493) radius 0.325
  circle A21 centre (6.4237, -1.2604) radius 0.325
  circle A22 centre (6.7131, -0.6595) radius 0.325
  line L5 (4.575, 0) -> (-1.425, 0) construction
  circle A23 centre (-1.425, 0) radius 2.8
  dimension "d15" = 16
  dimension "d16" = 11.75
  dimension "d17" = 4.475
  dimension "d18" = 0.65
  dimension "d20" = 360
  dimension "d21" = 6
  dimension "d22" = 5.6
  constraint midpoint L1 L4.start
  constraint perpendicular L1 L4
  constraint coincident L4.end A0.centre
  constraint coincident A1 A2.centre
  constraint parallel L4 L5
  constraint coincident L5.end A23.centre
  measures "d15" distance of L4.start L4.end
  measures "d16" diameter of A0
  measures "d17" diameter of A1
  measures "d18" diameter of A2
  measures "d21" distance of L4.end L5.end
  measures "d22" diameter of A23
extrude "Extrude4" add sketch "Sketch3" along normal blind 4.2 contours A0 A23 | A0 A23 | A0 A23 bodies 2
extrude "Extrude5" add 1 faces at (-4.6091, 0.2197, 22.75) along direction (0, 0, 1) blind 8.25 and the other way blind 22.75 separate body on bodies 2 makes body 3
extrude "Extrude6" cut 1 faces at (-4.6091, 0.2197, 0) along direction (0, 0, 1) blind 21 on bodies 3 bodies 3
sketch "Sketch4" plane through (0, 0, 0) normal (0, 0, 1) x (1, 0, 0)
  line L0 (0, 0) -> (-4.5, 0)
  dimension "d38" = 4.5
  constraint coincident L0.start origin
  constraint horizontal L0
  measures "d38" distance of L0.start L0.end
equation "d9 = -16.00 mm - 2.5 mm"
equation "d17 = 4.85 mm - ( 0.75 / 2 ) * 1 mm"
equation "d25 = 31 mm - 22.75 mm"
